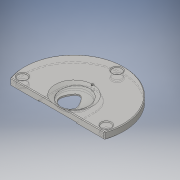
# Autodesk Inventor part: holder
Saved by Autodesk Inventor 2016 (Build 200138000, 138)
## iProperties
Created: 2018-05-23
Part Number: holder
Material: Generic
Document SubType Name: Modeling
Designer: Valued Customer
Density: 1 g/cm^3
Appearance: Default
Author: Valued Customer
Autodesk Inventor part; units mm, degrees
ref_plane "YZ Plane" through (0, 0, 0) normal (1, 0, 0) x (0, 1, 0)
ref_plane "Bottom Plane for Slope" through (0, 1.5, 0) normal (0, 1, 0) x (-1, 0, 0)
sketch "Bottom Plane" plane through (0, 1.5, 0) normal (0, 1, 0) x (-1, 0, 0)
  line L0 (-25.4, 25.4) -> (25.4, 25.4)
  line L1 (25.4, 25.4) -> (25.4, -25.4)
  line L2 (25.4, -25.4) -> (-25.4, -25.4)
  line L3 (-25.4, -25.4) -> (-25.4, 25.4)
  line L4 (-25.4, 25.4) -> (25.4, -25.4) construction
  line L5 (25.4, 25.4) -> (-25.4, -25.4) construction
  point P0 (0, 0)
  dimension "d26" = 50.8
  dimension "d27" = 50.8
  constraints: 12 end point, 2 midpoint, 2 parallel, 1 horizontal, 1 perpendicular
  measures "d26" distance of L1.end L2.end
  measures "d27" distance of L0.end L1.end
ref_plane "Top Plane for Slope" through (0, 4.5, 0) normal (0, 1, 0) x (-1, 0, 0)
sketch "Top Plane" plane through (0, 4.5, 0) normal (0, 1, 0) x (-1, 0, 0)
  line L0 (-25.4, 25.4) -> (25.4, 25.4)
  line L1 (25.4, 25.4) -> (25.4, -25.4)
  line L2 (25.4, -25.4) -> (-25.4, -25.4)
  line L3 (-25.4, -25.4) -> (-25.4, 25.4)
  line L4 (-25.4, 25.4) -> (25.4, -25.4) construction
  line L5 (25.4, 25.4) -> (-25.4, -25.4) construction
  point P0 (0, 0)
  dimension "d28" = 50.8
  dimension "d29" = 50.8
  constraints: 12 end point, 2 midpoint, 2 parallel, 1 horizontal, 1 perpendicular
  measures "d28" distance of L1.end L2.end
  measures "d29" distance of L0.end L1.end
ref_plane "Slope Plane" through (-25.4, 1.5, 25.4) normal (0.0589524, -0.9982608, 0) x (0, 0, -1)
sketch "master" plane through (0, 0, 0) normal (0, 1, 0) x (-1, 0, 0)
  circle A0 centre (0, 0) radius 36
  line L0 (0, 36) -> (0, -36) construction
  line L1 (12, -33.9411) -> (12, 33.9411)
  circle A1 centre (0, 0) radius 10 construction
  line L2 (10, 0) -> (12, 0) construction
  circle A2 centre (-1.7, 0) radius 13.7 construction
  line L3 (-36, 0) -> (12, 0) construction
  circle A3 centre (0, 0) radius 31 construction
  line L4 (7, -35.3129) -> (7, 35.3129) construction
  line L5 (0, 0) -> (-23.1404, -27.5776) construction
  line L6 (0, 0) -> (-23.1404, 27.5776) construction
  circle A4 centre (-1.7, 0) radius 11.7 construction
  line L7 (-1.7, -13.7) -> (-1.7, 13.7) construction
  line L8 (-1.7, -13.7) -> (12, -13.7) construction
  line L9 (-1.7, 13.7) -> (12, 13.7) construction
  point P0 (7, -30.1993)
  point P1 (7, 30.1993)
  point P2 (-19.9264, -23.7474)
  point P3 (-19.9264, 23.7474)
  point P4 (-31, 0)
  point P5 (0, -11.5758)
  point P6 (0, 11.5758)
  point P7 (-13.4, 0)
  dimension "d0" = 72
  dimension "d2" = 20
  dimension "d1" = 2
  dimension "d6" = 27.4
  dimension "d7" = 5
  dimension "d8" = 5
  dimension "d9" = 50
  dimension "d10" = 50
  dimension "d11" = 2
  constraints: 20 end point, 11 point on circle, 11 point on line, 5 coincident, 4 perpendicular, 3 centre point, 3 midpoint, 2 vertical, 1 horizontal, 1 horizontal alignment, 1 parallel, 1 tangent, 13 other
  measures "d1" distance of L2.start L2.end
  measures "d6" diameter of A2
  measures "d8" distance between parallel lines of L4 L1
  measures "d9" angle of L3 L5
  measures "d10" angle of L6 L3
  measures "d11" radial gap between concentric circles of A4 A2
extrude "Main Platform" add sketch "master" along normal blind 5 contours L1 A0 picked at (-3.9243, -1.3458)
sketch "Sketch3" plane through (0, 0, 0) normal (0, -1, 0) x (1, 0, 0)
  circle A0 centre (0, 0) radius 10 construction
  circle A1 centre (0, 0) radius 10
  constraints: 1 centre point, 1 coincident, 1 concentric
extrude "Main Hole" cut sketch "Sketch3" against normal blind 5
sketch "Sketch4" plane through (0, 0, 0) normal (0, -1, 0) x (1, 0, 0)
  circle A0 centre (1.7, 0) radius 13.7 construction
  circle A1 centre (1.7, 0) radius 13.7
  line L0 (1.7, 13.7) -> (-12, 13.7) construction
  line L1 (1.7, -13.7) -> (-12, -13.7) construction
  line L2 (-12, 13.7) -> (1.7, 13.7)
  line L3 (1.7, 13.7) -> (1.7, -13.7)
  line L4 (1.7, -13.7) -> (-12, -13.7)
  line L5 (-12, -13.7) -> (-12, 13.7)
  point P0 (0, 0)
  constraints: 8 end point, 2 parallel, 1 centre point, 1 coincident, 1 concentric, 1 horizontal, 1 perpendicular
extrude "Window Recess" cut sketch "Sketch4" against normal blind 1
sketch "Sketch5" plane through (0, 0, 0) normal (0, -1, 0) x (1, 0, 0)
  point P0 (0, 0)
  point P1 (13.4, 0)
hole "Window Removal Holes" at (13.4, 0, 0) direction (0, 1, 0) diameter 1.5 end through all
sketch "Sketch10" plane through (-25.4, 1.5, 25.4) normal (0.0589524, -0.9982608, 0) x (0, 0, -1)
  ellipse E0 centre (25.4, 27.0234) end of major axis (11.7, 27.0234) minor radius 13.6762 (39.1, 27.0234) -> (11.7, 27.0234) ccw construction
  line L0 (11.7, 13.3472) -> (11.7, 27.0234) construction
  line L1 (39.1, 27.0234) -> (39.1, 13.3472) construction
  ellipse E1 centre (25.4, 25.5622) end of major axis (35.4, 25.5622) minor radius 9.9826 construction
  line L2 (59.3411, 13.583) -> (-8.5411, 13.583) construction
  line L3 (39.1, 26.9644) -> (39.1, 13.2883) projected
  line L4 (39.1, 14.351) -> (11.7, 14.351)
  line L5 (11.7, 14.351) -> (11.7, 35.7061)
  line L6 (11.7, 35.7061) -> (39.1, 35.7061)
  line L7 (39.1, 35.7061) -> (39.1, 14.351)
  point P0 (25.4, 25.2674)
  constraints: 8 end point, 2 parallel, 1 horizontal, 1 perpendicular, 1 point on line, 2 other
extrude "Slope" add sketch "Sketch10" along normal blind 1
sketch "Sketch14" plane through (0, 0, 0) normal (0, -1, 0) x (1, 0, 0)
  point P0 (0, 0)
  point P1 (-7, 30.1993)
  point P2 (31, 0)
  point P3 (-7, -30.1993)
chamfer "Chamfer1" distance 2 angle 60 1 edges at (-10, 5, 0)
sketch "Sketch17" plane through (-25.4, 1.5, 25.4) normal (0.0589524, -0.9982608, 0) x (0, 0, -1)
  ellipse E0 centre (25.4, 25.4443) end of major axis (25.4, 15.4268) minor radius 10 (15.4, 25.4443) -> (35.4, 25.4443) ccw construction
  ellipse E1 centre (25.4, 26.4797) end of major axis (25.4, 36.6031) minor radius 10.0527 (35.4, 25.4443) -> (15.4, 25.4443) ccw construction
  ellipse E2 centre (25.4, 25.3852) end of major axis (25.4, 15.3678) minor radius 10 construction
  ellipse E3 centre (25.4, 25.4443) end of major axis (35.4, 25.4443) minor radius 9.9826 (15.4, 25.4443) -> (35.4, 25.4443) ccw construction
  line L0 (25.4, 35.4026) -> (32.7708, 19.5959) construction
  line L1 (25.4, 35.4026) -> (18.0292, 19.5959) construction
  line L2 (25.4, 35.4026) -> (25.4, 19.5959) construction
  line L3 (32.7708, 19.5959) -> (18.0292, 19.5959) construction
  line L4 (28.184, 29.4323) -> (22.616, 29.4323) construction
  line L5 (58.9857, 14.0822) -> (-8.1857, 14.0822) construction
  line L6 (-8.1857, 14.0822) -> (-8.1857, 35.4026) construction
  line L7 (-8.1857, 35.4026) -> (58.9857, 35.4026) construction
  line L8 (58.9857, 35.4026) -> (58.9857, 14.0822) construction
  spline S0 degree 5 poles (25.4, 29.4323) (26.7138, 29.432) (28.9448, 27.9113) (31.9512, 21.8517) (32.9232, 20.462) (25.6746, 12.422) (16.6165, 20.5026) (19.1302, 21.7816) (21.8974, 27.8954) (24.0775, 29.4325) (25.4, 29.4323) knots 0 0 0 0 0 0 0.199988 0.334999 0.499228 0.663457 0.798679 1 1 1 1 1 1
  line L9 (30.5619, 24.333) -> (20.2381, 24.333) construction
  line L10 (25.4, 19.5959) -> (25.4, 13.3472) construction
  line L11 (39.1, 13.3472) -> (11.7, 13.3472) projected
  point P0 (25.4, 25.2674)
  point P1 (25.4, 15.9117)
  point P2 (19.2424, 19.5959)
  dimension "d81" = 25
  dimension "d82" = 25
  constraints: 22 end point, 7 point on line, 4 midpoint, 3 parallel, 2 coincident, 2 horizontal, 1 perpendicular, 1 vertical, 1 vertical alignment, 11 other
  measures "d81" angle of L2 L0
  measures "d82" angle of L2 L1
extrude "Extrusion6" cut sketch "Sketch17" along normal through all
sketch "Sketch15" plane through (0, 5, 0) normal (0, 1, 0) x (1, 0, 0)
  point P0 (0, 0)
  point P1 (31, 0)
  point P2 (-7, -30.1993)
  point P3 (-7, 30.1993)
hole "Top Magnet Holes" at (-7, 5, -30.1993) at (31, 5, 0) at (-7, 5, 30.1993) direction (0, -1, 0) diameter 6.5 depth 0.5
hole "Bottom Magnet Holes" at (-7, 0, 30.1993) at (31, 0, 0) at (-7, 0, -30.1993) direction (0, 1, 0) diameter 6.5 depth 1.5
chamfer "Chamfer7" distance 0.5 angle 45 1 edges at (-12, 2.5, 33.9411)
chamfer "Chamfer8" distance 0.5 angle 45 1 edges at (-12, 2.5, -33.9411)
chamfer "Chamfer9" distance 0.5 angle 45 1 edges at (-12, 5, -19.7735)
chamfer "Chamfer10" distance 0.5 angle 45 1 edges at (-12, 5, 19.7735)
chamfer "Chamfer11" distance 0.5 angle 45 1 edges at (-12, 0, 23.5706)
chamfer "Chamfer12" distance 0.5 angle 45 1 edges at (-12, 0, -23.5706)
chamfer "Chamfer13" distance 0.5 angle 45 1 edges at (36, 5, 0)
chamfer "Chamfer14" distance 0.5 angle 45 1 edges at (36, 0, 0)
chamfer "Chamfer15" distance 0.5 angle 45 1 edges at (-7, 5, -33.4493)
chamfer "Chamfer16" distance 0.5 angle 45 1 edges at (31, 5, -3.25)
chamfer "Chamfer17" distance 0.5 angle 45 1 edges at (-7, 5, 26.9493)
chamfer "Chamfer18" distance 0.5 angle 45 1 edges at (-7, 0, 33.4493)
chamfer "Chamfer19" distance 0.5 angle 45 1 edges at (31, 0, 3.25)
chamfer "Chamfer20" distance 0.5 angle 45 1 edges at (-7, 0, -26.9493)
body "Solid1"
